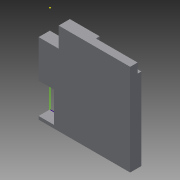
# Autodesk Inventor part: Prototype1
Saved by Autodesk Inventor 2015 (Build 190159000, 159)
## iProperties
Created: 2015-03-15
Part Number: Prototype1
Material: Generic
Document SubType Name: Modeling
Designer: Jesse
Density: 1 g/cm^3
Appearance: Default
Author: Jesse
Autodesk Inventor part; units mm, degrees
ref_plane "YZ Plane" through (0, 0, 0) normal (1, 0, 0) x (0, 1, 0)
ref_plane "XZ Plane" through (0, 0, 0) normal (0, 1, 0) x (-1, 0, 0)
ref_plane "XY Plane" through (0, 0, 0) normal (0, 0, 1) x (1, 0, 0)
sketch "Sketch1" plane through (0, 0, 0) normal (0, 1, 0) x (-1, 0, 0)
  line L0 (12.5, 12.5) -> (-12.5, 12.5)
  line L1 (-12.5, 12.5) -> (-12.5, -12.5)
  line L2 (-12.5, -12.5) -> (12.5, -12.5)
  line L3 (12.5, -12.5) -> (12.5, 12.5)
  line L4 (57.15, 6) -> (31.15, 6)
  line L5 (31.15, 6) -> (31.15, -6)
  line L6 (31.15, -6) -> (57.15, -6)
  line L7 (57.15, -6) -> (57.15, 6)
  line L8 (-31.15, 6) -> (-57.15, 6)
  line L9 (-57.15, 6) -> (-57.15, -6)
  line L10 (-57.15, -6) -> (-31.15, -6)
  line L11 (-31.15, -6) -> (-31.15, 6)
  line L12 (9.55, 55.15) -> (-9.55, 55.15)
  line L13 (-9.55, 55.15) -> (-9.55, 36.05)
  line L14 (-9.55, 36.05) -> (9.55, 36.05)
  line L15 (9.55, 36.05) -> (9.55, 55.15)
  line L16 (9.55, -36.05) -> (-9.55, -36.05)
  line L17 (-9.55, -36.05) -> (-9.55, -55.15)
  line L18 (-9.55, -55.15) -> (9.55, -55.15)
  line L19 (9.55, -55.15) -> (9.55, -36.05)
  line L20 (57.15, 57.15) -> (-57.15, 57.15)
  line L21 (-57.15, 57.15) -> (-57.15, -57.15)
  line L22 (-57.15, -57.15) -> (57.15, -57.15)
  line L23 (57.15, -57.15) -> (57.15, 57.15)
  circle A0 centre (-28.575, -28.575) radius 16.0636
  line L24 (-28.575, -28.575) -> (-44.6386, -28.575)
  line L25 (-28.575, -28.575) -> (-20.5432, -42.4865)
  line L26 (-28.575, -28.575) -> (-12.5114, -28.575) construction
  line L27 (-28.575, -28.575) -> (-20.5432, -14.6635)
  circle A1 centre (-24.5591, -21.6193) radius 3.2
  circle A2 centre (-24.5591, -35.5307) radius 3.2
  circle A3 centre (-36.6068, -28.575) radius 3.2
  line L28 (0, 0) -> (-12.5, -12.5)
  circle A4 centre (-28.575, 28.575) radius 16.0636
  line L29 (-28.575, 28.575) -> (-44.6386, 28.575)
  line L30 (-28.575, 28.575) -> (-20.5432, 14.6635)
  line L31 (-28.575, 28.575) -> (-20.5432, 42.4865)
  circle A5 centre (-24.5591, 35.5307) radius 3.2
  circle A6 centre (-24.5591, 21.6193) radius 3.2
  circle A7 centre (-36.6068, 28.575) radius 3.2
  circle A8 centre (28.575, 28.575) radius 16.0636
  line L32 (28.575, 28.575) -> (12.5114, 28.575)
  line L33 (28.575, 28.575) -> (36.6068, 14.6635)
  line L34 (28.575, 28.575) -> (36.6068, 42.4865)
  circle A9 centre (32.5909, 35.5307) radius 3.2
  circle A10 centre (32.5909, 21.6193) radius 3.2
  circle A11 centre (20.5432, 28.575) radius 3.2
  circle A12 centre (28.575, -28.575) radius 16.0636
  line L35 (28.575, -28.575) -> (12.5114, -28.575)
  line L36 (28.575, -28.575) -> (36.6068, -42.4865)
  line L37 (28.575, -28.575) -> (36.6068, -14.6635)
  circle A13 centre (32.5909, -21.6193) radius 3.2
  circle A14 centre (32.5909, -35.5307) radius 3.2
  circle A15 centre (20.5432, -28.575) radius 3.2
  line L38 (34.1909, 38.302) -> (36.6068, 42.4865)
  line L39 (30.9909, 32.7595) -> (28.575, 28.575)
  line L40 (30.9909, 24.3905) -> (28.575, 28.575)
  line L41 (34.1909, 18.848) -> (36.6068, 14.6635)
  line L42 (23.7432, 28.575) -> (28.575, 28.575)
  line L43 (17.3432, 28.575) -> (12.5114, 28.575)
  line L44 (28.575, 28.575) -> (23.7432, 28.575)
  line L45 (-28.575, 28.575) -> (-26.1591, 24.3905)
  line L46 (-22.9591, 18.848) -> (-20.5432, 14.6635)
  line L47 (-26.1591, 32.7595) -> (-28.575, 28.575)
  line L48 (-22.9591, 38.302) -> (-20.5432, 42.4865)
  line L49 (-39.8068, 28.575) -> (-44.6386, 28.575)
  line L50 (-33.4068, 28.575) -> (-28.575, 28.575)
  line L51 (-22.9591, 18.848) -> (-20.5432, 14.6635)
  line L52 (-44.6386, -28.575) -> (-39.8068, -28.575)
  line L53 (-33.4068, -28.575) -> (-28.575, -28.575)
  line L54 (-28.575, -28.575) -> (-26.1591, -32.7595)
  line L55 (-22.9591, -38.302) -> (-20.5432, -42.4865)
  line L56 (-28.575, -28.575) -> (-26.1591, -24.3905)
  line L57 (-22.9591, -18.848) -> (-20.5432, -14.6635)
  line L58 (0, 0) -> (0, -57.15)
  line L59 (0, 0) -> (-57.15, 0)
  line L60 (0, 0) -> (-31.15, 0)
  line L61 (0, 0) -> (0, -36.05)
  line L62 (0, 0) -> (0, -12.5)
  line L63 (0, 0) -> (-12.5, 0)
  line L64 (-57.15, 0) -> (-57.15, -6)
  line L65 (-57.15, 0) -> (-57.15, -57.15)
  line L66 (-57.15, -57.15) -> (0, -57.15)
  line L67 (0, -55.15) -> (0, -57.15)
  line L68 (0, -36.05) -> (0, -55.15)
  line L69 (0, -36.05) -> (0, -12.5)
  point P0 (-28.575, 28.575)
  point P1 (28.575, 28.575)
  point P2 (28.575, -28.575)
  dimension "d2" = 25
  dimension "d3" = 25
  dimension "d4" = 12.5
  dimension "d5" = 12.5
  dimension "d6" = 6
  dimension "d7" = 12
  dimension "d8" = 26
  dimension "d9" = 26
  dimension "d10" = 6
  dimension "d11" = 12
  dimension "d12" = 19.1
  dimension "d13" = 19.1
  dimension "d14" = 9.55
  dimension "d15" = 19.1
  dimension "d16" = 19.1
  dimension "d17" = 9.55
  dimension "d22" = 0
  dimension "d23" = 0
  dimension "d24" = 2
  dimension "d25" = 2
  dimension "d26" = 114.3
  dimension "d28" = 57.15
  dimension "d29" = 57.15
  dimension "d30" = 114.3
  dimension "d37" = 28.575
  dimension "d38" = 28.575
  dimension "d39" = 6.4
  dimension "d40" = 6.4
  dimension "d41" = 6.4
  dimension "d43" = 120
  dimension "d44" = 120
  dimension "d45" = 32.1272
  dimension "d46" = 28.575
  dimension "d47" = 28.575
  dimension "d48" = 28.575
  dimension "d49" = 28.575
  dimension "d50" = 28.575
  dimension "d51" = 28.575
  dimension "d52" = 6.4
  dimension "d53" = 6.4
  dimension "d54" = 6.4
  dimension "d55" = 120
  dimension "d56" = 120
  dimension "d57" = 32.1272
  dimension "d58" = 6.4
  dimension "d59" = 6.4
  dimension "d60" = 6.4
  dimension "d61" = 120
  dimension "d62" = 120
  dimension "d63" = 32.1272
  dimension "d64" = 6.4
  dimension "d65" = 6.4
  dimension "d66" = 6.4
  dimension "d67" = 120
  dimension "d68" = 120
  dimension "d69" = 32.1272
  constraints: 140 end point, 30 point on circle, 23 point on line, 19 collinear, 19 midpoint, 16 centre point, 12 parallel, 11 horizontal, 6 perpendicular, 1 equal length
  measures "d2" distance of L2.end L0.start
  measures "d3" distance of L0.start L0.end
  measures "d4" distance from line of L28.start L0
  measures "d5" distance from line of L3 L28.start
  measures "d6" distance from line of L6 L28.start
  measures "d7" distance between parallel lines of L6 L4
  measures "d8" distance of L4.start L4.end
  measures "d9" distance of L10.end L9.end
  measures "d10" distance from line of L10 L28.start
  measures "d11" distance between parallel lines of L10 L8
  measures "d12" distance of L14.end L12.start
  measures "d13" distance of L12.start L12.end
  measures "d14" distance from line of L15 L28.start
  measures "d15" distance of L17.end L18.end
  measures "d16" distance of L18.end L16.start
  measures "d17" distance from line of L28.start L19
  measures "d22" distance between parallel lines of L7 L23
  measures "d23" distance between parallel lines of L21 L9
  measures "d24" distance between parallel lines of L20 L12
  measures "d25" distance between parallel lines of L22 L18
  measures "d26" distance between parallel lines of L21 L23
  measures "d28" distance from line of L21 L28.start
  measures "d29" distance from line of L20 L28.start
  measures "d30" distance of L22.end L20.start
  measures "d37" distance from line of L21 L24.start
  measures "d38" distance from line of L22 L24.start
  measures "d39" diameter of A1
  measures "d40" diameter of A2
  measures "d41" diameter of A3
  measures "d43" angle of L24 L25
  measures "d44" angle of L27 L25
  measures "d45" diameter of A0
  measures "d46" distance from line of L21 point (-28.575, 28.575)
  measures "d47" distance from line of L20 point (-28.575, 28.575)
  measures "d48" distance from line of L23 point (28.575, 28.575)
  measures "d49" distance from line of L20 point (28.575, 28.575)
  measures "d50" distance from line of L23 point (28.575, -28.575)
  measures "d51" distance from line of L22 point (28.575, -28.575)
  measures "d52" diameter of A5
  measures "d53" diameter of A6
  measures "d54" diameter of A7
  measures "d55" angle of L29 L30
  measures "d56" angle of L31 L30
  measures "d57" diameter of A4
  measures "d58" diameter of A9
  measures "d59" diameter of A10
  measures "d60" diameter of A11
  measures "d61" angle of L32 L33
  measures "d62" angle of L34 L33
  measures "d63" diameter of A8
  measures "d64" diameter of A13
  measures "d65" diameter of A14
  measures "d66" diameter of A15
  measures "d67" angle of L35 L36
  measures "d68" angle of L37 L36
  measures "d69" diameter of A12
extrude "Extrusion1" add sketch "Sketch1" along normal blind 7 contours L1 L2 L58 L16 L17 L18 L22 L21 L10 L11 L59 | A0 L25 A2 L27 A1 | L27 A1 L24 A3 A0 | A0 L24 A3 L25 A2
sketch "Sketch2" plane through (0, 0, 0) normal (0, -1, 0) x (1, 0, 0)
  circle A0 centre (36.6068, -28.575) radius 3.2 projected
  circle A1 centre (36.6068, -28.575) radius 3.2
  circle A2 centre (24.5591, -21.6193) radius 3.2 projected
  circle A3 centre (24.5591, -21.6193) radius 3.2
  circle A4 centre (24.5591, -35.5307) radius 3.2 projected
  circle A5 centre (24.5591, -35.5307) radius 3.2
  point P0 (0, 0)
  constraints: 3 centre point, 3 coincident
extrude "Extrusion2" add sketch "Sketch2" against normal blind 2
sketch "Sketch3" plane through (0, 0, 0) normal (0, -1, 0) x (1, 0, 0)
  line L0 (31.15, -6) -> (57.15, -6)
  line L1 (57.15, -6) -> (57.15, 0)
  line L2 (57.15, 0) -> (31.15, 0)
  line L3 (31.15, 0) -> (31.15, -6)
  point P0 (0, 0)
  constraints: 8 end point, 2 parallel, 1 horizontal, 1 perpendicular
extrude "Extrusion3" add sketch "Sketch3" against normal blind 4.65
sketch "Sketch4" plane through (0, 7, 0) normal (0, 1, 0) x (1, 0, 0)
  line L0 (9.55, 55.15) -> (0, 55.15)
  line L1 (0, 55.15) -> (0, 36.05)
  line L2 (0, 36.05) -> (9.55, 36.05)
  line L3 (9.55, 36.05) -> (9.55, 55.15)
  point P0 (0, 0)
  constraints: 8 end point, 2 parallel, 1 horizontal, 1 perpendicular
body "Solid1"
